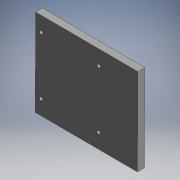
# Autodesk Inventor part: Part14
Saved by Autodesk Inventor 2016 (Build 200138000, 138)
## iProperties
Created: 2018-01-18
Part Number: Part14
Material: Generic
Document SubType Name: Modeling
Designer: student
Density: 1 g/cm^3
Appearance: Default
Author: student
Autodesk Inventor part; units mm, degrees
ref_plane "YZ Plane" through (0, 0, 0) normal (1, 0, 0) x (0, 1, 0)
ref_plane "XZ Plane" through (0, 0, 0) normal (0, 1, 0) x (-1, 0, 0)
ref_plane "XY Plane" through (0, 0, 0) normal (0, 0, 1) x (1, 0, 0)
sketch "Sketch1" plane through (0, 0, 0) normal (0, 0, 1) x (1, 0, 0)
  circle A0 centre (0.2751, 52.8541) radius 1.4214
  circle A1 centre (53.1386, 52.6394) radius 1.4214
  circle A2 centre (52.924, -0.224) radius 1.4214
  circle A3 centre (0.0605, -0.0094) radius 1.4214
  circle A4 centre (0.2751, 52.8541) radius 1.4214
  circle A5 centre (0.0605, -0.0094) radius 1.4214
  circle A6 centre (52.924, -0.224) radius 1.4214
  circle A7 centre (53.1386, 52.6394) radius 1.4214
  line L0 (-5.2979, -23.5291) -> (88.6821, -23.9107)
  line L1 (88.6821, -23.9107) -> (89.0881, 76.0893)
  line L2 (89.0881, 76.0893) -> (-4.8919, 76.4709)
  line L3 (-4.8919, 76.4709) -> (-5.2979, -23.5291)
  line L4 (-5.2979, -23.5291) -> (2.9514, -23.54) construction
  circle A8 centre (26.5572, 26.3424) radius 11 construction
  circle A9 centre (41.9941, 10.7796) radius 1.5 construction
  circle A10 centre (10.9944, 10.9055) radius 1.5 construction
  circle A11 centre (11.1202, 41.9052) radius 1.5 construction
  circle A12 centre (42.12, 41.7793) radius 1.5 construction
  circle A13 centre (0.2148, 52.8996) radius 1.4224 construction
  circle A14 centre (0, 0) radius 1.4224 construction
  circle A15 centre (52.8996, -0.2148) radius 1.4224 construction
  circle A16 centre (53.1143, 52.6848) radius 1.4224 construction
  line L5 (-5.3215, -5.2784) -> (58.178, -5.5363) construction
  line L6 (58.178, -5.5363) -> (58.4358, 57.9632) construction
  line L7 (58.4358, 57.9632) -> (-5.0637, 58.221) construction
  line L8 (-5.0637, 58.221) -> (-5.3215, -5.2784) construction
  line L9 (88.8851, 26.0893) -> (-5.1926, 26.4713) construction
  point P0 (0.0605, -0.0094)
  point P1 (88.9156, 66.1637)
  dimension "d7" = 100
  dimension "d8" = 93.98
  constraints: 12 end point, 8 centre point, 4 parallel, 2 midpoint, 1 other
  measures "d7" vertical distance of L0.end L1.end
  measures "d8" horizontal distance of L1.end L2.end
extrude "Extrusion1" add sketch "Sketch1" along normal blind 6.35
sketch "Sketch2" plane through (0, 0, 6.35) normal (0, 0, 1) x (1, 0, 0)
  circle A0 centre (0.0605, -0.0094) radius 1.4214 construction
  circle A1 centre (52.924, -0.224) radius 1.4214 construction
  circle A2 centre (53.1386, 52.6394) radius 1.4214 construction
  circle A3 centre (0.2751, 52.8541) radius 1.4214 construction
  line L0 (-5.2979, -23.5291) -> (88.6821, -23.9107) construction
  line L1 (89.0881, 76.0893) -> (-4.8919, 76.4709) construction
  line L2 (-4.8919, 76.4709) -> (-5.2979, -23.5291) construction
  line L3 (89.0881, 76.0893) -> (89.043, 64.9782)
  line L4 (89.043, 64.9782) -> (82.693, 65.004)
  line L5 (82.693, 65.004) -> (82.6479, 53.8929)
  line L6 (82.6479, 53.8929) -> (88.9978, 53.8671)
  line L7 (89.043, 64.9782) -> (88.9978, 53.8671)
  line L8 (88.9979, 53.8673) -> (88.9527, 42.7562)
  line L9 (88.9527, 42.7562) -> (82.6028, 42.782)
  line L10 (82.6028, 42.782) -> (82.5577, 31.6709)
  line L11 (82.5577, 31.6709) -> (88.9076, 31.6451)
  line L12 (88.9527, 42.7562) -> (88.9076, 31.6451)
  line L13 (88.9076, 31.6453) -> (88.8625, 20.5341)
  line L14 (88.8625, 20.5341) -> (82.5126, 20.5599)
  line L15 (82.5126, 20.5599) -> (82.4675, 9.4488)
  line L16 (82.4675, 9.4488) -> (88.8174, 9.423)
  line L17 (88.8625, 20.5341) -> (88.8174, 9.423)
  line L18 (88.8174, 9.4232) -> (88.7723, -1.6879)
  line L19 (88.7723, -1.6879) -> (82.4223, -1.6621)
  line L20 (82.4223, -1.6621) -> (82.3772, -12.7732)
  line L21 (82.3772, -12.7732) -> (88.7272, -12.799)
  line L22 (88.7723, -1.6879) -> (88.7272, -12.799)
  point P0 (0, 0)
  dimension "d12" = 6.35
  dimension "d14" = 11.1111
  dimension "d31" = 22.2222
  constraints: 40 end point, 4 centre point, 4 perpendicular, 1 collinear, 30 other
  measures "d12" distance of L3.end L4.end
  measures "d14" vertical distance of L4.end L5.end
  measures "d31" distance of L3.end L8.end
extrude "Extrusion2" cut sketch "Sketch2" against normal blind 25.4
equation "\"d14\" = d11"
equation "\"d11\" = 11.111111"
body "Solid1"
